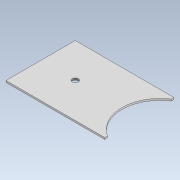
# Autodesk Inventor part: platina_1
Saved by Autodesk Inventor 2021 (Build 250183000, 183)
## iProperties
Created: 2021-04-25
Part Number: platina_1
Material: Genérico
Document SubType Name: Modeling
Designer: j2seb
Density: 1 g/cm^3
Appearance: Valor por defecto
Author: j2seb
Autodesk Inventor part; units mm, degrees
ref_plane "YZ Plane" through (0, 0, 0) normal (1, 0, 0) x (0, 1, 0)
ref_plane "XZ Plane" through (0, 0, 0) normal (0, 1, 0) x (-1, 0, 0)
ref_plane "XY Plane" through (0, 0, 0) normal (0, 0, 1) x (1, 0, 0)
sketch "Boceto1" plane through (0, 0, 0) normal (0, 1, 0) x (-1, 0, 0)
  line L0 (0, 0) -> (0, -40)
  line L1 (0, -40) -> (60, -40)
  line L2 (60, 0) -> (0, 0)
  line L3 (60, -40) -> (60, 0)
  dimension "d1" = 60
  dimension "d3" = 40
  constraints: 8 end point, 2 vertical, 1 horizontal, 1 parallel, 1 vertical alignment
  measures "d1" distance of L0.end L1.end
  measures "d3" distance of L0.start L0.end
extrude "Extrusión1" add sketch "Boceto1" along normal blind 1
sketch "Boceto2" plane through (0, 0, 0) normal (0, -1, 0) x (1, 0, 0)
  line L0 (0, 0) -> (0, -40) projected
  circle A0 centre (9, -20) radius 22
  point P0 (0, -20)
  dimension "d7" = 44
  dimension "d8" = 9
  constraints: 1 centre point, 1 horizontal alignment, 1 midpoint
  measures "d7" diameter of A0
  measures "d8" distance from line of A0.centre L0
extrude "Extrusión2" cut sketch "Boceto2" against normal through all
sketch "Boceto3" plane through (0, 1, 0) normal (0, 1, 0) x (1, 0, 0)
  arc A0 (-0.1652, 40) -> (-0.1652, 0) centre (9, 20) ccw projected
  line L0 (-0.1652, 40) -> (-60, 40) projected
  line L1 (-60, 40) -> (-60, 0) projected
  line L2 (-60, 0) -> (-0.1652, 0) projected
  line L3 (-60, 40) -> (-3, 40)
  line L4 (-3, 40) -> (-3, 0)
  line L5 (-3, 0) -> (-60, 0)
  line L6 (-60, 0) -> (-60, 40)
  point P0 (0, 0)
  point P1 (-3, 38.4391)
  point P2 (-3, 1.5609)
  dimension "d11" = 57
  constraints: 8 end point, 2 parallel, 1 horizontal, 1 perpendicular, 1 point on line
  measures "d11" distance between parallel lines of L1 L4
extrude "Extrusión3" cut sketch "Boceto3" against normal through all contours A0 L4 L2 L1 L0 keep common part
sketch "Boceto4" plane through (0, 0, 0) normal (0, -1, 0) x (1, 0, 0)
  point P0 (-40, -20)
hole "Agujero1" at (-40, 0, -20) direction (0, 1, 0) diameter 3.4 end through all
